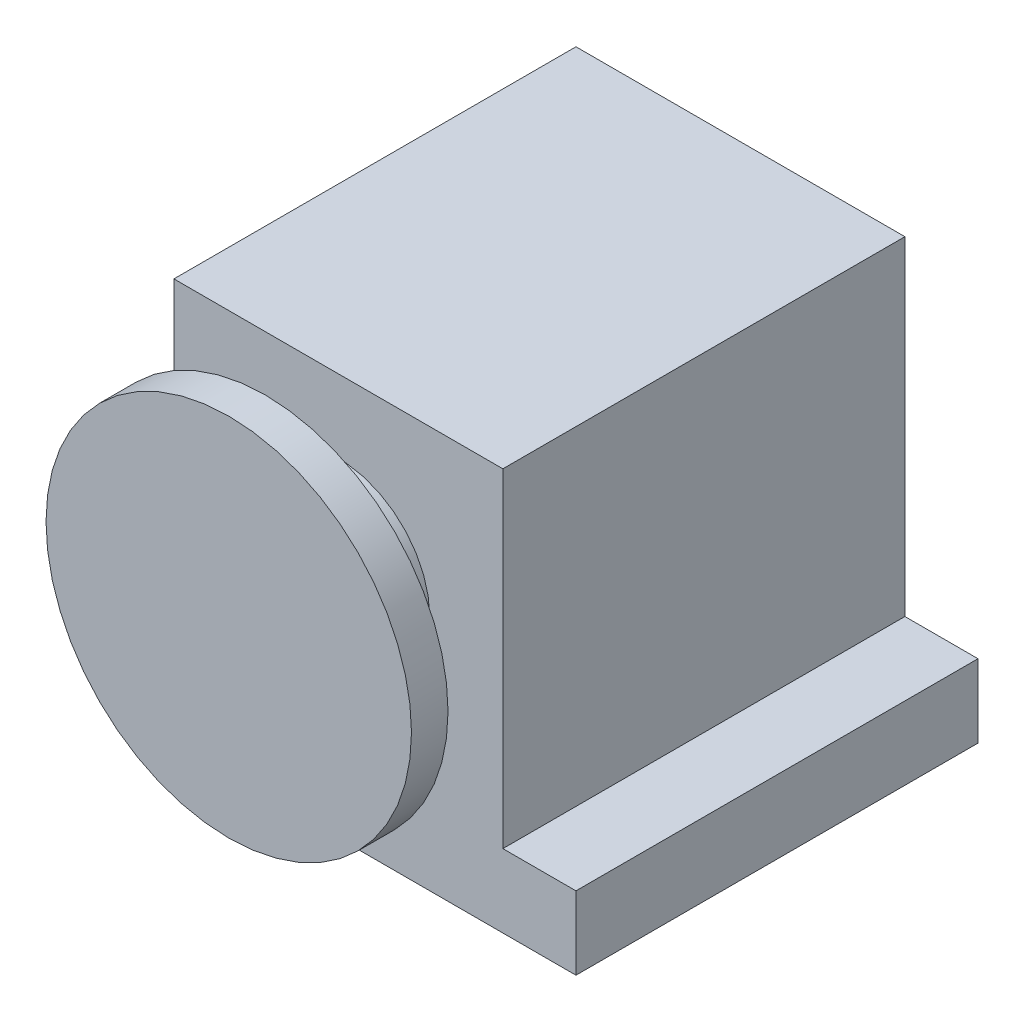
# Autodesk Inventor part: A_Gearbox
Saved by Autodesk Inventor 2023 (Build 270158000, 158)
## iProperties
Created: 2024-08-24
Part Number: A_Gearbox
Material: Generic
Document SubType Name: Modeling
Designer: think
Density: 1 g/cm^3
Appearance: Default
Author: think
Autodesk Inventor part; units mm, degrees
ref_plane "YZ Plane" through (0, 0, 0) normal (1, 0, 0) x (0, 1, 0)
ref_plane "XZ Plane" through (0, 0, 0) normal (0, 1, 0) x (-1, 0, 0)
ref_plane "XY Plane" through (0, 0, 0) normal (0, 0, 1) x (1, 0, 0)
sketch "Sketch1" plane through (0, 0, 0) normal (0, 0, 1) x (1, 0, 0)
  line L0 (0, 0) -> (0, 20)
  line L1 (0, 20) -> (20, 20)
  line L2 (20, 20) -> (20, 110)
  line L3 (20, 110) -> (110, 110)
  line L4 (110, 110) -> (110, 20)
  line L5 (110, 20) -> (130, 20)
  line L6 (130, 20) -> (130, 0)
  line L7 (130, 0) -> (0, 0)
  dimension "d0" = 20
  dimension "d1" = 110
  dimension "d2" = 90
  dimension "d3" = 130
  constraints: 16 end point, 6 perpendicular, 2 point on line, 1 collinear, 1 vertical
  measures "d0" distance of L5.end L6.end
  measures "d1" distance between parallel lines of L7 L3
  measures "d2" distance of L2.end L3.end
  measures "d3" distance of L6.end L0.start
extrude "Extrusion1" add sketch "Sketch1" along normal blind 110
sketch "Sketch2" plane through (0, 0, 110) normal (0, 0, 1) x (1, 0, 0)
  line L0 (110, 110) -> (20, 110) projected
  line L1 (0, 0) -> (130, 0) projected
  circle A0 centre (65, 65) radius 25
  line L2 (65, 65) -> (65, 0) construction
  line L3 (0, 0) -> (130, 0) construction
  dimension "d6" = 65
  dimension "d7" = 50
  constraints: 2 end point, 1 centre point, 1 midpoint, 1 vertical
  measures "d6" distance of L2.start L2.end
  measures "d7" diameter of A0
extrude "Extrusion2" add sketch "Sketch2" along normal blind 20
sketch "Sketch3" plane through (65, 65, 130) normal (0, 0, 1) x (1, 0, 0)
  circle A0 centre (0, 0) radius 50
  circle A1 centre (0, 0) radius 25 projected
  point P0 (-65, -65)
  dimension "d10" = 100
  constraints: 1 centre point, 1 concentric
  measures "d10" diameter of A0
extrude "Extrusion3" add sketch "Sketch3" along normal blind 10 contours A0 | A1
body "Solid1"
